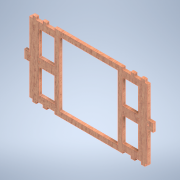
# Autodesk Inventor part: DoorFrameFront_V2
Saved by Autodesk Inventor 2022.2 (Build 262287000, 287)
## iProperties
Created: 2023-03-04
Part Number: DoorFrameFront_V2
Material: Wood (Oak)
Document SubType Name: Modeling
Designer: jaege
Density: 0.76 g/cm^3
Appearance: Red Oak - Natural Low Gloss
Author: jaege
Autodesk Inventor part; units mm, degrees
ref_plane "YZ Plane" through (0, 0, 0) normal (1, 0, 0) x (0, 1, 0)
ref_plane "XZ Plane" through (0, 0, 0) normal (0, 1, 0) x (-1, 0, 0)
ref_plane "XY Plane" through (0, 0, 0) normal (0, 0, 1) x (1, 0, 0)
sketch "Sketch1" plane through (0, 0, 0) normal (0, 0, 1) x (1, 0, 0)
  line L0 (45, -50) -> (-45, -50)
  line L1 (-45, -50) -> (-45, 50)
  line L2 (-45, 50) -> (45, 50)
  line L3 (45, 50) -> (45, -50)
  line L4 (45, -50) -> (-45, 50) construction
  line L5 (-45, -50) -> (45, 50) construction
  line L6 (53, 58) -> (-53, 58)
  line L7 (-53, 58) -> (-53, 54.5)
  line L8 (-53, -58) -> (53, -58)
  line L9 (53, -58) -> (53, -54.5)
  line L10 (-20, 50) -> (20, 50)
  line L11 (-20, -50) -> (20, -50)
  line L12 (-45, -20) -> (-45, 20)
  line L13 (45, -20) -> (45, 20)
  line L14 (-53, 6.5) -> (-77, 6.5)
  line L15 (-100, 6.5) -> (-100, -6.5)
  line L16 (-100, -6.5) -> (-92, -6.5)
  line L17 (-53, -6.5) -> (-53, 6.5) construction
  line L18 (-53, 0) -> (53, 0)
  circle A0 centre (-92, 0) radius 1.45
  circle A1 centre (-77, 0) radius 1.45
  line L19 (0, 50) -> (0, -50)
  line L20 (-53, 6.5) -> (-53, -6.5) construction
  line L21 (-53, -6.5) -> (-53, -44.5)
  line L22 (53, 6.5) -> (53, 44.5)
  line L23 (53, -6.5) -> (53, 6.5) construction
  line L24 (-92, -6.5) -> (-77, -6.5) construction
  line L25 (-77, -6.5) -> (-77, -44.5)
  line L26 (-77, -58) -> (-92, -58) construction
  line L27 (-92, -58) -> (-92, -54.5) construction
  line L28 (-92, -58) -> (-77, -58) construction
  line L29 (-77, -58) -> (-77, -58.5) construction
  line L30 (-77, -58.5) -> (-81.5, -58.5) construction
  line L31 (-92, -58.5) -> (-92, -58) construction
  line L32 (-92, -54.5) -> (-87.5, -54.5)
  line L33 (-87.5, -54.5) -> (-87.5, -58.5)
  line L34 (-81.5, -58.5) -> (-81.5, -54.5)
  line L35 (-81.5, -54.5) -> (-77, -54.5)
  line L36 (-77, 6.5) -> (-77, 44.5)
  line L37 (-77, 58) -> (-92, 58) construction
  line L38 (-92, 58) -> (-92, 54.5) construction
  line L39 (-92, 58) -> (-77, 58) construction
  line L40 (-77, 58) -> (-77, 58.5) construction
  line L41 (-77, 58.5) -> (-81.5, 58.5) construction
  line L42 (-92, 58.5) -> (-92, 58) construction
  line L43 (-92, 54.5) -> (-87.5, 54.5)
  line L44 (-87.5, 54.5) -> (-87.5, 58.5)
  line L45 (-81.5, 58.5) -> (-81.5, 54.5)
  line L46 (-81.5, 54.5) -> (-77, 54.5)
  line L47 (-77, 6.5) -> (-92, 6.5) construction
  line L48 (-92, 6.5) -> (-100, 6.5)
  line L49 (-92, -6.5) -> (-77, -6.5) construction
  line L50 (-77, -6.5) -> (-53, -6.5)
  line L51 (-77, 54.5) -> (-77, 58) construction
  line L52 (-92, 54.5) -> (-92, 6.5)
  line L53 (-87.5, 58.5) -> (-92, 58.5) construction
  line L54 (-81.5, 58.5) -> (-87.5, 58.5)
  line L55 (-92, -54.5) -> (-92, -6.5)
  line L56 (-87.5, -58.5) -> (-92, -58.5) construction
  line L57 (-81.5, -58.5) -> (-87.5, -58.5)
  line L58 (-77, -54.5) -> (-77, -58) construction
  line L59 (-77, 54.5) -> (-71.5, 54.5)
  line L60 (-53, 54.5) -> (-53, 44.5) construction
  line L61 (-53, 44.5) -> (-77, 44.5)
  line L62 (-77, 44.5) -> (-77, 54.5) construction
  line L63 (-77, -54.5) -> (-71.5, -54.5)
  line L64 (-53, -54.5) -> (-53, -54)
  line L65 (-53, -44.5) -> (-77, -44.5)
  line L66 (-77, -44.5) -> (-77, -54.5) construction
  line L67 (-71.5, 54.5) -> (-65.5, 54.5) construction
  line L68 (-65.5, 54.5) -> (-65.5, 58.5)
  line L69 (-65.5, 58.5) -> (-71.5, 58.5)
  line L70 (-71.5, 58.5) -> (-71.5, 54.5)
  line L71 (-71.5, -54.5) -> (-65.5, -54.5) construction
  line L72 (-65.5, -54.5) -> (-65.5, -58.5)
  line L73 (-65.5, -58.5) -> (-71.5, -58.5)
  line L74 (-71.5, -58.5) -> (-71.5, -54.5)
  line L75 (-71.5, 54.5) -> (-65.5, 54.5) construction
  line L76 (-65.5, 54.5) -> (-53, 54.5)
  line L77 (-77, 44.5) -> (-77, 54.5) construction
  line L78 (-53, 44.5) -> (-53, 6.5)
  line L79 (-53, 54.5) -> (-53, 44.5) construction
  line L80 (-77, -44.5) -> (-77, -54.5) construction
  line L81 (-53, -44.5) -> (-53, -54.5) construction
  line L82 (-53, -54) -> (-53, -44.5) construction
  line L83 (-65.5, -54.5) -> (-53, -54.5)
  line L84 (-71.5, -54.5) -> (-65.5, -54.5) construction
  line L85 (-53, -54.5) -> (-53, -58)
  line L86 (53, 6.5) -> (77, 6.5)
  line L87 (100, 6.5) -> (100, -6.5)
  line L88 (100, -6.5) -> (92, -6.5)
  circle A2 centre (92, 0) radius 1.45
  circle A3 centre (77, 0) radius 1.45
  line L89 (92, -6.5) -> (77, -6.5) construction
  line L90 (77, -6.5) -> (77, -44.5)
  line L91 (77, -58) -> (92, -58) construction
  line L92 (92, -58) -> (92, -54.5) construction
  line L93 (92, -58) -> (77, -58) construction
  line L94 (77, -58) -> (77, -58.5) construction
  line L95 (77, -58.5) -> (81.5, -58.5) construction
  line L96 (92, -58.5) -> (92, -58) construction
  line L97 (92, -54.5) -> (87.5, -54.5)
  line L98 (87.5, -54.5) -> (87.5, -58.5)
  line L99 (81.5, -58.5) -> (81.5, -54.5)
  line L100 (81.5, -54.5) -> (77, -54.5)
  line L101 (92, 54.5) -> (87.5, 54.5)
  line L102 (92, 58) -> (92, 54.5) construction
  line L103 (77, 6.5) -> (77, 44.5)
  line L104 (81.5, 54.5) -> (77, 54.5)
  line L105 (77, 58) -> (92, 58) construction
  line L106 (92, 58) -> (77, 58) construction
  line L107 (77, 58) -> (77, 58.5) construction
  line L108 (77, 58.5) -> (81.5, 58.5) construction
  line L109 (81.5, 58.5) -> (81.5, 54.5)
  line L110 (92, 58.5) -> (92, 58) construction
  line L111 (87.5, 54.5) -> (87.5, 58.5)
  line L112 (77, 6.5) -> (92, 6.5) construction
  line L113 (92, 6.5) -> (100, 6.5)
  line L114 (92, -6.5) -> (77, -6.5) construction
  line L115 (77, -6.5) -> (53, -6.5)
  line L116 (77, 54.5) -> (77, 58) construction
  line L117 (92, 54.5) -> (92, 6.5)
  line L118 (87.5, 58.5) -> (92, 58.5) construction
  line L119 (81.5, 58.5) -> (87.5, 58.5)
  line L120 (92, -54.5) -> (92, -6.5)
  line L121 (87.5, -58.5) -> (92, -58.5) construction
  line L122 (81.5, -58.5) -> (87.5, -58.5)
  line L123 (77, -54.5) -> (77, -58) construction
  line L124 (77, 54.5) -> (71.5, 54.5)
  line L125 (53, 44.5) -> (77, 44.5)
  line L126 (77, 44.5) -> (77, 54.5) construction
  line L127 (77, -54.5) -> (71.5, -54.5)
  line L128 (53, -44.5) -> (77, -44.5)
  line L129 (77, -44.5) -> (77, -54.5) construction
  line L130 (71.5, 54.5) -> (65.5, 54.5) construction
  line L131 (65.5, 54.5) -> (65.5, 58.5)
  line L132 (65.5, 58.5) -> (71.5, 58.5)
  line L133 (71.5, 58.5) -> (71.5, 54.5)
  line L134 (71.5, -54.5) -> (65.5, -54.5) construction
  line L135 (65.5, -54.5) -> (65.5, -58.5)
  line L136 (65.5, -58.5) -> (71.5, -58.5)
  line L137 (71.5, -58.5) -> (71.5, -54.5)
  line L138 (71.5, 54.5) -> (65.5, 54.5) construction
  line L139 (65.5, 54.5) -> (53, 54.5)
  line L140 (77, 44.5) -> (77, 54.5) construction
  line L141 (77, -44.5) -> (77, -54.5) construction
  line L142 (65.5, -54.5) -> (53, -54.5)
  line L143 (71.5, -54.5) -> (65.5, -54.5) construction
  line L144 (53, 44.5) -> (53, 54.5) construction
  line L145 (53, 54.5) -> (53, 58)
  line L146 (53, -44.5) -> (53, -6.5)
  line L147 (53, -54.5) -> (53, -44.5) construction
  point P0 (0, 0)
  point P1 (0, 54)
  point P2 (0, 0)
  point P3 (-49, 0)
  point P4 (0, 0)
  point P5 (-53, 0)
  point P6 (0, 0)
  point P7 (0, 0)
  point P8 (-84.5, -58)
  point P9 (-84.5, 58)
  point P10 (-65, 44.5)
  point P11 (-81.5, 56.5)
  point P12 (-71.5, 56.5)
  point P13 (84.5, -58)
  point P14 (84.5, 58)
  point P15 (65, 44.5)
  point P16 (81.5, 56.5)
  point P17 (71.5, 56.5)
  dimension "d0" = 100
  dimension "d1" = 90
  dimension "d2" = 8
  dimension "d9" = 13
  dimension "d10" = 47
  dimension "d11" = 2.9
  dimension "d12" = 15
  dimension "d13" = 24
  dimension "d16" = 15
  dimension "d17" = 0.5
  dimension "d18" = 6
  dimension "d19" = 4.5
  dimension "d20" = 4.5
  dimension "d21" = 4
  dimension "d24" = 10
  dimension "d25" = 10
  dimension "d27" = 10
  dimension "d28" = 6
  dimension "d29" = 8
  dimension "d30" = 8
  dimension "d31" = 4.5
  constraints: 296 end point, 87 parallel, 62 symmetric about line, 29 perpendicular, 16 horizontal, 14 midpoint, 12 point on line, 7 horizontal alignment, 4 centre point, 4 vertical alignment, 1 collinear, 1 equal radius, 3 other
  measures "d0" distance of L0.end L1.end
  measures "d1" distance of L1.end L2.end
  measures "d2" distance between parallel lines of L2 L6
  measures "d9" distance of L15.start L15.end
  measures "d10" distance of L14.start L15.start
  measures "d11" diameter of A0
  measures "d12" distance of A1.centre A0.centre
  measures "d13" distance from line of L7 A1.centre
  measures "d16" distance of L26.start L26.end
  measures "d17" distance of L26.start L29.end
  measures "d18" distance between parallel lines of L34 L33
  measures "d19" distance of L34.end L35.end
  measures "d20" distance of L27.end L32.end
  measures "d21" distance of L32.end L33.end
  measures "d24" distance from line of point (-65, 44.5) L59
  measures "d25" distance between parallel lines of L65 L63
  measures "d27" distance of L73.end L30.end
  measures "d28" distance of L72.end L73.end
  measures "d29" distance between parallel lines of L1 L21
  measures "d30" distance between parallel lines of L3 L22
  measures "d31" distance between parallel lines of L2 L76
extrude "Extrusion1" add sketch "Sketch1" along normal blind 4
body "Solid1"
